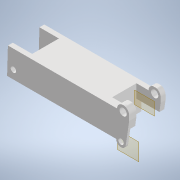
# Autodesk Inventor part: Dedo_1
Saved by Autodesk Inventor 2020 (Build 240168000, 168)
## iProperties
Created: 2021-07-22
Part Number: Dedo_1
Material: Generic
Document SubType Name: Modeling
Designer: chalo
Density: 1 g/cm^3
Appearance: Default
Author: chalo
Autodesk Inventor part; units mm, degrees
ref_plane "YZ Plane" through (0, 0, 0) normal (1, 0, 0) x (0, 1, 0)
ref_plane "XZ Plane" through (0, 0, 0) normal (0, 1, 0) x (-1, 0, 0)
ref_plane "XY Plane" through (0, 0, 0) normal (0, 0, 1) x (1, 0, 0)
ref_plane "Work Plane1" through (-21.75, 2.25, -0.6) normal (0, 0, 1) x (-1, 0, 0)
ref_plane "Work Plane2" through (-30.217, -5.375, 6) normal (0, 0, 1) x (1, 0, 0)
sketch "Sketch1" plane through (-30.217, -5.375, 6) normal (0, 0, 1) x (1, 0, 0)
  circle A0 centre (2.6155, -1.0303) radius 1.1 projected
  circle A1 centre (3.467, 10) radius 1.5 projected
  line L0 (4.6155, -1.0303) -> (5.967, 8)
  line L1 (0.6155, -1.0303) -> (-44.3845, -1.0303)
  arc A2 (0.6155, -1.0303) -> (4.6155, -1.0303) centre (2.6155, -1.0303) ccw
  line L2 (5.967, 8) -> (5.967, 10)
  line L3 (0.967, 10) -> (-44.033, 10)
  arc A3 (5.967, 10) -> (0.967, 10) centre (3.467, 10) ccw
  line L4 (-44.033, 10) -> (-44.3845, -1.0303)
  point P0 (30.217, 5.375)
  dimension "d0" = 2
  dimension "d1" = 2
  dimension "d2" = 2
  dimension "d3" = 2.5
  dimension "d4" = 2
  dimension "d5" = 2.5
  dimension "d6" = 2.5
  dimension "d7" = 45
  dimension "d8" = 45
  constraints: 10 end point, 4 horizontal alignment, 4 point on circle, 2 centre point, 2 horizontal, 1 vertical
  measures "d0" distance of L0.start A0.centre
  measures "d1" distance of A0.centre L1.start
  measures "d2" radius of A2
  measures "d3" horizontal distance of A1.centre L0.end
  measures "d4" distance of L0.end L2.end
  measures "d5" distance of A1.centre L3.start
  measures "d6" radius of A3
  measures "d7" distance of L3.start L3.end
  measures "d8" distance of L1.start L1.end
extrude "Extrusion1" add sketch "Sketch1" along normal blind 1
sketch "Sketch2" plane through (-30.217, -5.375, 6) normal (0, 0, -1) x (-1, 0, 0)
  arc A0 (-0.967, 10) -> (-5.967, 10) centre (-3.467, 10) ccw projected
  line L0 (-5.967, 8) -> (-5.967, 10) projected
  line L1 (-4.6155, -1.0303) -> (-5.967, 8) projected
  arc A1 (-4.6155, -1.0303) -> (-0.6155, -1.0303) centre (-2.6155, -1.0303) ccw projected
  line L2 (44.3845, -1.0303) -> (-0.6155, -1.0303) projected
  line L3 (44.033, 10) -> (44.3845, -1.0303) projected
  line L4 (-0.967, 10) -> (44.033, 10) projected
  circle A2 centre (-2.6155, -1.0303) radius 1.1 projected
  circle A3 centre (-3.467, 10) radius 1.5 projected
  line L5 (44.3845, -1.0303) -> (-0.6155, -1.0303) projected
  line L6 (4.033, -1.0303) -> (4.033, 10)
  line L7 (-0.967, 10) -> (44.033, 10) projected
  point P0 (-30.217, 5.375)
  point P1 (4.033, 10)
  point P2 (4.033, -1.0303)
  dimension "d11" = 5
  constraints: 2 end point, 2 point on line, 1 perpendicular
  measures "d11" distance from line of L4.start L6
extrude "Extrusion2" add sketch "Sketch2" along normal blind 14 contours L4 L3 L2 L6
sketch "Sketch3" plane through (-30.217, -5.375, -8) normal (0, 0, -1) x (-1, 0, 0)
  circle A0 centre (-3.467, 10) radius 1.5 projected
  line L0 (-8.467, 7.625) -> (-8.467, 12.375) projected
  line L1 (-8.467, 7.625) -> (-0.967, 7.625) projected
  line L2 (-0.967, 12.375) -> (-0.967, 7.625) projected
  line L3 (-8.467, 12.375) -> (-0.967, 12.375) projected
  line L4 (44.033, 10) -> (4.033, 10) projected
  line L5 (4.033, 10) -> (4.033, -1.0303) projected
  line L6 (4.033, -1.0303) -> (44.3845, -1.0303) projected
  line L7 (44.3845, -1.0303) -> (44.033, 10) projected
  circle A1 centre (-3.467, 10) radius 1.5 projected
  circle A2 centre (-2.6155, -1.0303) radius 1.1 projected
  line L8 (4.033, -1.0303) -> (4.033, 10) projected
  line L9 (-0.967, 10) -> (4.033, 10) projected
  arc A3 (-0.967, 10) -> (-5.967, 10) centre (-3.467, 10) ccw projected
  line L10 (-5.967, 8) -> (-5.967, 10) projected
  line L11 (-4.6155, -1.0303) -> (-5.967, 8) projected
  arc A4 (-4.6155, -1.0303) -> (-0.6155, -1.0303) centre (-2.6155, -1.0303) ccw projected
  line L12 (4.033, -1.0303) -> (-0.6155, -1.0303) projected
  line L13 (4.033, 10) -> (4.033, -1.0303) projected
  line L14 (4.033, 4.4849) -> (-5.4409, 4.4849)
  line L15 (-4.6155, -1.0303) -> (-5.967, 8) projected
  point P0 (-30.217, 5.375)
  point P1 (-5.4409, 4.4849)
  point P2 (-2.6863, 12.375)
  point P3 (-4.2476, 12.375)
  constraints: 2 end point, 1 horizontal, 1 midpoint, 1 point on line
extrude "Extrusion3" add sketch "Sketch3" against normal blind 2 contours L11 L10 A3 L3 L2 L1 | L1 L2 L9 L5 L14 L11
sketch "Sketch4" plane through (-30.217, -5.375, 6) normal (0, 0, -1) x (-1, 0, 0)
  circle A0 centre (-3.467, 10) radius 1.5 projected
  circle A1 centre (-2.6155, -1.0303) radius 1.1 projected
  line L0 (4.033, -1.0303) -> (4.033, 10) projected
  line L1 (-0.967, 10) -> (4.033, 10) projected
  arc A2 (-0.967, 10) -> (-5.967, 10) centre (-3.467, 10) ccw projected
  line L2 (-5.967, 8) -> (-5.967, 10) projected
  line L3 (-4.6155, -1.0303) -> (-5.967, 8) projected
  arc A3 (-4.6155, -1.0303) -> (-0.6155, -1.0303) centre (-2.6155, -1.0303) ccw projected
  line L4 (4.033, -1.0303) -> (-0.6155, -1.0303) projected
  circle A4 centre (-3.467, 10) radius 1.5 projected
  circle A5 centre (-3.467, 10) radius 2.5
  arc A6 (-0.967, 10) -> (-5.967, 10) centre (-3.467, 10) ccw projected
  circle A7 centre (-3.467, 10) radius 1.5 projected
  line L5 (44.033, 10) -> (-0.967, 10) projected
  arc A8 (-0.967, 10) -> (-2.6863, 12.375) centre (-3.467, 10) ccw projected
  line L6 (-2.6863, 12.375) -> (-4.2476, 12.375) projected
  arc A9 (-4.2476, 12.375) -> (-5.967, 10) centre (-3.467, 10) ccw projected
  line L7 (-5.967, 10) -> (-5.967, 8) projected
  line L8 (-5.967, 8) -> (-5.4409, 4.4849) projected
  line L9 (-5.4409, 4.4849) -> (4.033, 4.4849) projected
  line L10 (4.033, 4.4849) -> (4.033, -1.0303) projected
  line L11 (4.033, -1.0303) -> (44.3845, -1.0303) projected
  line L12 (44.3845, -1.0303) -> (44.033, 10) projected
  point P0 (-30.217, 5.375)
  constraints: 1 centre point, 1 coincident, 1 concentric
extrude "Extrusion4" add sketch "Sketch4" along normal blind 2 contours L9 L3 L2 A5 L1 L0 | A5 A2 L6
sketch "Sketch5" plane through (-74.25, 4.625, 7) normal (0, 1, 0) x (1, 0, 0)
  line L0 (45, 3) -> (45, 0) projected
  line L1 (40, 3) -> (45, 3) projected
  line L2 (40, 3) -> (40, 13) projected
  line L3 (45, 13) -> (40, 13) projected
  line L4 (45, 15) -> (45, 13) projected
  line L5 (0, 15) -> (45, 15) projected
  line L6 (0, 15) -> (0, 0) projected
  line L7 (45, 0) -> (0, 0) projected
  line L8 (8, 13) -> (-0.5, 13)
  line L9 (-0.5, 13) -> (-0.5, 2)
  line L10 (-0.5, 2) -> (8, 2)
  line L11 (8, 2) -> (8, 13)
  point P0 (74.25, 7)
  point P1 (8, 7.5)
  point P2 (0, 7.5)
  dimension "d18" = 8
  dimension "d19" = 0.5
  dimension "d20" = 2
  constraints: 8 end point, 2 midpoint, 2 parallel, 1 horizontal, 1 horizontal alignment, 1 perpendicular
  measures "d18" distance between parallel lines of L11 L6
  measures "d19" distance between parallel lines of L6 L9
  measures "d20" distance between parallel lines of L7 L10
extrude "Extrusion5" cut sketch "Sketch5" against normal blind 9 contours L10 L9 L8 L6 | L6 L8 L11 L10
shell "Shell1" thickness 1 removed faces 1 at (-61.1509, -6.4053, 1.6667)
sketch "Sketch6" plane through (-30.217, -5.375, 7) normal (0, 0, 1) x (1, 0, 0)
  circle A0 centre (-41.7707, 2.5) radius 1.1
  line L0 (-44.033, 10) -> (-44.3845, -1.0303) construction
  point P0 (30.217, 5.375)
  point P1 (-44.3198, 1)
  dimension "d24" = 2.2
  dimension "d25" = 1.5
  dimension "d26" = 2.5
  constraints: 1 centre point
  measures "d24" diameter of A0
  measures "d25" vertical distance of point (-44.32, 1) A0.centre
  measures "d26" distance from line of L0 A0.centre
extrude "Extrusion6" cut sketch "Sketch6" against normal up to surface (2 mm away)
body "Solid1"
